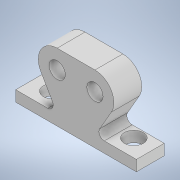
# Autodesk Inventor part: montaz_wachlarzy_2
Saved by Autodesk Inventor 2022 (Build 260153000, 153)
## iProperties
Created: 2022-12-26
Part Number: montaz_wachlarzy_2
Material: Generic
Document SubType Name: Modeling
Designer: Kamil
Density: 1 g/cm^3
Appearance: Default
Author: Kamil
Autodesk Inventor part; units mm, degrees
ref_plane "YZ Plane" through (0, 0, 0) normal (1, 0, 0) x (0, 1, 0)
ref_plane "XZ Plane" through (0, 0, 0) normal (0, 1, 0) x (-1, 0, 0)
ref_plane "XY Plane" through (0, 0, 0) normal (0, 0, 1) x (1, 0, 0)
sketch "Sketch1" plane through (0, 0, 0) normal (0, 0, 1) x (1, 0, 0)
  line L0 (28.1525, 7.6) -> (28.1525, 11.1) projected
  line L1 (-46.8475, 11.1) -> (28.1525, 11.1) projected
  line L2 (-46.8475, 11.1) -> (-46.8475, 7.6) projected
  line L3 (-46.8475, 7.6) -> (-22.3475, 7.6) projected
  line L4 (-22.3475, 0) -> (-22.3475, 7.6) projected
  line L5 (-22.3475, 0) -> (-18.695, 0) projected
  line L6 (-18.695, 0) -> (-18.695, 2.6) projected
  line L7 (-15, 2.6) -> (-18.695, 2.6) projected
  line L8 (-15, 0) -> (-15, 2.6) projected
  line L9 (-15, 0) -> (-3.695, 0) projected
  line L10 (-3.695, 0) -> (-3.695, 2.6) projected
  line L11 (0, 2.6) -> (-3.695, 2.6) projected
  line L12 (0, 0) -> (0, 2.6) projected
  line L13 (0, 0) -> (3.6525, 0) projected
  line L14 (3.6525, 0) -> (3.6525, 7.6) projected
  line L15 (3.6525, 7.6) -> (28.1525, 7.6) projected
  line L16 (-24.3475, 7.6) -> (-24.3475, 11.1) projected
  line L17 (5.6525, 7.6) -> (5.6525, 11.1) projected
  line L18 (-3.5975, 2.6) -> (-3.5975, 11.1)
  line L19 (-0.0975, 2.6) -> (-0.0975, 11.1)
  line L20 (-15.0975, 2.6) -> (-15.0975, 11.1)
  line L21 (-18.5975, 2.6) -> (-18.5975, 11.1)
  line L22 (-59.3475, 18.1) -> (-59.3475, 7.1) projected
  line L23 (-59.3475, 7.1) -> (-53.3475, 7.1) projected
  line L24 (-53.3475, 7.1) -> (-53.3475, 8.1) projected
  line L25 (-53.3475, 8.1) -> (-53.3475, 11.1) projected
  line L26 (-53.3475, 11.1) -> (-53.3475, 18.1) projected
  line L27 (-53.3475, 18.1) -> (-59.3475, 18.1) projected
  line L28 (-18.5975, 11.1) -> (-0.0975, 11.1)
  line L29 (-0.0975, 11.1) -> (-0.0975, 18.1)
  line L30 (-0.0975, 18.1) -> (-18.5975, 18.1)
  line L31 (-18.5975, 18.1) -> (-18.5975, 11.1)
  line L32 (-53.3475, 18.1) -> (10.0147, 18.1)
  circle A0 centre (-9.3475, 18.1) radius 3.5
  circle A1 centre (-9.3475, 18.1) radius 1.75
  line L33 (1.8262, 11.1) -> (-20.5213, 11.1)
  line L34 (-20.5213, 11.1) -> (-20.5213, 13.1)
  line L35 (-20.5213, 13.1) -> (-14.8475, 13.1)
  line L36 (1.8262, 13.1) -> (1.8262, 11.1)
  line L37 (-12.8475, 18.1) -> (-12.8475, 15.1)
  line L38 (-5.8475, 18.1) -> (-5.8475, 15.1)
  arc A2 (-14.8475, 13.1) -> (-12.8475, 15.1) centre (-14.8475, 15.1) ccw
  line L39 (-3.8475, 13.1) -> (1.8262, 13.1)
  arc A3 (-5.8475, 15.1) -> (-3.8475, 13.1) centre (-3.8475, 15.1) ccw
  point P0 (-5.8475, 13.1)
  dimension "d0" = 7
  dimension "d1" = 3.5
  dimension "d2" = 2
  dimension "d3" = 2
  dimension "d4" = 2
  constraints: 32 end point, 6 point on circle, 6 point on line, 6 tangent, 5 parallel, 4 centre point, 4 perpendicular, 4 vertical, 3 horizontal, 1 coincident, 10 other
  measures "d0" diameter of A0
  measures "d1" diameter of A1
  measures "d2" distance of L33.end L34.end
  measures "d3" radius of A2
  measures "d4" radius of A3
ref_plane "Work Plane1" through (-24.3475, 0, -5.16) normal (0, 0, -1) x (0, 1, 0)
extrude "Extrusion1" add sketch "Sketch1" against normal up to surface (5.16 mm away) contours L1 L29 L39 L36 | L1 L31 L35 A2 L37 A0 L38 A3 L39 L29 | L1 L34 L35 L31 | A0 L30 A1 | L30 A1 A0
sketch "Sketch2" plane through (-20.5213, 11.1, 0) normal (0, -1, 0) x (1, 0, 0)
  circle A0 centre (18.6738, -3.2) radius 1.75 projected
  circle A1 centre (3.6738, -3.2) radius 1.75 projected
  line L0 (-3.8262, -10.16) -> (-1.3262, -10.16) projected
  arc A2 (-1.3262, -10.16) -> (-1.3262, -5.16) centre (-1.3262, -7.66) ccw projected
  line L1 (-1.3262, -5.16) -> (-3.8262, -5.16) projected
  line L2 (-3.8262, -5.16) -> (-3.8262, -10.16) projected
  line L3 (23.6738, -10.16) -> (26.1738, -10.16) projected
  line L4 (26.1738, -10.16) -> (26.1738, -5.16) projected
  line L5 (26.1738, -5.16) -> (23.6738, -5.16) projected
  arc A3 (23.6738, -5.16) -> (23.6738, -10.16) centre (23.6738, -7.66) ccw projected
  line L6 (48.6738, 0) -> (48.6738, -46.6121) projected
  line L7 (48.6738, -46.6121) -> (26.0339, -46.6121) projected
  line L8 (26.0339, -46.6121) -> (26.0339, -30.5552) projected
  line L9 (26.0339, -30.5552) -> (14.0514, -9.5814) projected
  line L10 (14.0514, -9.5814) -> (8.2961, -9.5814) projected
  line L11 (8.2961, -9.5814) -> (-3.8262, -30.8) projected
  line L12 (-3.8262, -30.8) -> (-3.8262, -46.6121) projected
  line L13 (-3.8262, -46.6121) -> (-26.3262, -46.6121) projected
  line L14 (-26.3262, -46.6121) -> (-26.3262, 0) projected
  line L15 (-26.3262, 0) -> (48.6738, 0) projected
  line L16 (22.3475, -5.16) -> (16.6738, -5.16) projected
  line L17 (16.6738, 0) -> (16.6738, -5.16) projected
  line L18 (22.3475, 0) -> (16.6738, 0) projected
  line L19 (22.3475, 0) -> (22.3475, -5.16) projected
  circle A4 centre (3.6738, -3.2) radius 1.75 projected
  line L20 (5.6738, -5.16) -> (0, -5.16) projected
  line L21 (0, 0) -> (0, -5.16) projected
  line L22 (5.6738, 0) -> (0, 0) projected
  line L23 (5.6738, 0) -> (5.6738, -5.16) projected
  circle A5 centre (18.6738, -3.2) radius 1.75 projected
  circle A6 centre (3.6738, -3.2) radius 1.75 projected
  line L24 (14.0514, -9.5814) -> (22.3475, -5.16)
  line L25 (0, 0) -> (0, -5.16) projected
  line L26 (0, -5.16) -> (8.2961, -9.5814)
  point P0 (20.5213, 0)
  constraints: 4 end point
extrude "Extrusion2" add sketch "Sketch2" against normal up to surface (2 mm away) contours L17 L16 L24 L10 L26 L20 L23 L15
sketch "Sketch3" plane through (-20.5213, 11.1, 0) normal (0, -1, 0) x (1, 0, 0)
  circle A0 centre (3.6738, -3.2) radius 1.75 projected
  circle A1 centre (18.6738, -3.2) radius 1.75 projected
  point P0 (20.5213, 0)
extrude "Extrusion3" cut sketch "Sketch3" against normal blind 10
fillet "Fillet1" radius 2 1 edges at (-9.3475, 13.1, -5.16)
sketch "Sketch4" plane through (-3.8475, 13.1, 0) normal (0, 1, 0) x (1, 0, 0)
  line L0 (-11, 0) -> (-11, 7.16) projected
  line L1 (0, 7.16) -> (-11, 7.16) projected
  line L2 (0, 0) -> (0, 7.16) projected
  line L3 (5.6738, 0) -> (0, 0) projected
  line L4 (5.6738, 0) -> (5.6738, 5.16) projected
  line L5 (-2.6223, 9.5814) -> (5.6738, 5.16) projected
  line L6 (-8.3777, 9.5814) -> (-2.6223, 9.5814) projected
  line L7 (-16.6738, 5.16) -> (-8.3777, 9.5814) projected
  line L8 (-16.6738, 0) -> (-16.6738, 5.16) projected
  line L9 (-11, 0) -> (-16.6738, 0) projected
  circle A0 centre (-13, 3.2) radius 1.75 projected
  circle A1 centre (2, 3.2) radius 1.75 projected
  line L10 (2, 3.2) -> (5.2, 3.2)
  line L11 (-8.3777, 9.5814) -> (-2.6223, 9.5814) projected
  line L12 (-5.5, 9.5814) -> (-5.5, 7.6751)
  line L13 (5.2, 1.3525) -> (2, -0.495)
  line L14 (2, -0.495) -> (-1.2, 1.3525)
  line L15 (-1.2, 1.3525) -> (-1.2, 5.0475)
  line L16 (-1.2, 5.0475) -> (2, 6.895)
  line L17 (2, 6.895) -> (5.2, 5.0475)
  line L18 (5.2, 5.0475) -> (5.2, 1.3525)
  line L19 (-13, 3.2) -> (-16.2, 3.2)
  line L20 (-16.2, 5.0475) -> (-13, 6.895)
  line L21 (-13, 6.895) -> (-9.8, 5.0475)
  line L22 (-9.8, 5.0475) -> (-9.8, 1.3525)
  line L23 (-9.8, 1.3525) -> (-13, -0.495)
  line L24 (-13, -0.495) -> (-16.2, 1.3525)
  line L25 (-16.2, 1.3525) -> (-16.2, 5.0475)
  line L26 (-9, 0) -> (-9, 5.16) projected
  line L27 (-2, 0) -> (-2, 5.16) projected
  line L28 (0, 0) -> (0, 7.16) projected
  line L29 (-2.174, 0.4287) -> (0, 0.4287)
  line L30 (0, 0.4287) -> (0, 7.16)
  line L31 (0, 7.16) -> (-2.174, 7.16)
  line L32 (-2.174, 7.16) -> (-2.174, 0.4287)
  line L33 (0, 7.16) -> (-11, 7.16) projected
  line L34 (-11, 0) -> (-9, 0)
  line L35 (-9, 0) -> (-9, 7.16)
  line L36 (-9, 7.16) -> (-11, 7.16)
  line L37 (-11, 7.16) -> (-11, 0)
  line L38 (-2, 0) -> (-2, 5.16) projected
  line L39 (0, 0) -> (-2, 0) projected
  line L40 (0, 0) -> (0, 7.16) projected
  line L41 (-2, 5.16) -> (0, 7.16) projected
  line L42 (-11, 0) -> (-11, 7.16) projected
  line L43 (-9, 0) -> (-11, 0) projected
  line L44 (-9, 0) -> (-9, 5.16) projected
  line L45 (-11, 7.16) -> (-9, 5.16) projected
  point P0 (3.8475, 0)
  point P1 (-2, 0)
  point P2 (-2.174, 7.16)
  point P3 (-2, 0.4287)
  dimension "d12" = 3.2
  constraints: 46 end point, 4 parallel, 3 horizontal, 3 midpoint, 2 coincident, 2 perpendicular, 2 symmetric about line, 1 point on line, 1 vertical, 26 other
  measures "d12" distance of L10.start L10.end
extrude "Extrusion4" cut sketch "Sketch4" along normal blind 10 contours L0 L23 L22 L21 L45 L26 L34 | L0 L21 L22 L23 | L45 L1 L35 | L1 L41 L27 L29 L32 | L2 L16 L15 L14 L29 L27 L41 | L2 L14 L15 L16 | L29 L2 L39 L27
sketch "Sketch5" plane through (-5.8475, 13.1, 0) normal (0, 1, 0) x (1, 0, 0)
  line L0 (-0.174, 7.16) -> (-7, 7.16) projected
  line L1 (-0.174, 7.16) -> (-0.174, 0.4287) projected
  line L2 (-0.174, 0.4287) -> (0, 0.4287) projected
  line L3 (0, 0.4287) -> (0, 0) projected
  line L4 (7.6738, 0) -> (0, 0) projected
  line L5 (7.6738, 0) -> (7.6738, 5.16) projected
  line L6 (-0.6223, 9.5814) -> (7.6738, 5.16) projected
  line L7 (-6.3777, 9.5814) -> (-0.6223, 9.5814) projected
  line L8 (-14.6738, 5.16) -> (-6.3777, 9.5814) projected
  line L9 (-14.6738, 0) -> (-14.6738, 5.16) projected
  line L10 (-7, 0) -> (-14.6738, 0) projected
  line L11 (-7, 0) -> (-7, 7.16) projected
  circle A0 centre (-11, 3.2) radius 1.75 projected
  circle A1 centre (4, 3.2) radius 1.75 projected
  line L12 (0, 0) -> (0, 0.4287) projected
  line L13 (-14.6738, 0) -> (7.6738, 0) projected
  line L14 (0, 0.4287) -> (-0.174, 0.4287)
  line L15 (-0.174, 0.4287) -> (-0.174, 0)
  line L16 (-0.174, 0) -> (0, 0)
  line L17 (0, 0) -> (0, 0.4287)
  point P0 (5.8475, 0)
  constraints: 8 end point, 2 parallel, 1 horizontal, 1 perpendicular, 1 point on line
extrude "Extrusion5" cut sketch "Sketch5" along normal blind 10 contours L2 L3 L13 L15
sketch "Sketch6" plane through (0, 0, 0) normal (0, 0, 1) x (1, 0, 0)
  line L0 (-6.0216, 13.1) -> (-6.0216, 19.1899) projected
  arc A0 (-6.0216, 19.1899) -> (-12.8475, 18.1) centre (-9.3475, 18.1) ccw projected
  line L1 (-12.8475, 18.1) -> (-12.8475, 13.1) projected
  line L2 (-12.8475, 13.1) -> (-20.5213, 13.1) projected
  line L3 (-20.5213, 13.1) -> (-20.5213, 11.1) projected
  line L4 (-20.5213, 11.1) -> (1.8262, 11.1) projected
  line L5 (1.8262, 11.1) -> (1.8262, 13.1) projected
  line L6 (1.8262, 13.1) -> (-6.0216, 13.1) projected
  circle A1 centre (-9.3475, 18.1) radius 1.75 projected
  line L7 (-59.3475, 18.1) -> (-59.3475, 7.1) projected
  line L8 (-59.3475, 7.1) -> (-53.3475, 7.1) projected
  line L9 (-53.3475, 7.1) -> (-53.3475, 8.1) projected
  line L10 (-53.3475, 8.1) -> (-53.3475, 11.1) projected
  line L11 (-53.3475, 11.1) -> (-53.3475, 18.1) projected
  line L12 (-53.3475, 18.1) -> (-59.3475, 18.1) projected
  line L13 (-9.3475, 18.1) -> (-9.3475, 20.1)
  circle A2 centre (-9.3475, 20.1) radius 1.75
  circle A3 centre (-9.3475, 20.1) radius 3.5
  line L14 (-6.4698, 13.1) -> (1.8262, 13.1) projected
  line L15 (-12.8475, 20.1) -> (-5.8475, 20.1)
  line L16 (-5.8475, 20.1) -> (-5.8475, 13.1)
  line L17 (-5.8475, 13.1) -> (-12.8475, 13.1)
  line L18 (-12.8475, 13.1) -> (-12.8475, 20.1)
  point P0 (0, 0)
  point P1 (-12.8475, 18.1)
  dimension "d17" = 2
  constraints: 10 end point, 2 coincident, 2 parallel, 1 centre point, 1 horizontal, 1 perpendicular, 1 point on line, 1 vertical, 3 other
  measures "d17" distance of L13.start L13.end
extrude "Extrusion6" add sketch "Sketch6" against normal up to surface (5.16 mm away) contours L14 L17 L1 A0 A3 A1 L0 | L0 A3 L16 L6 | A3 A1 A2 L15 A0 L0 | L0 A0 L15 A3 | A3 A1 A2 | A1 A3 | L15 A0 A2 A3 | L15 A2 A0 | A3 A0 L15 A2 A1 | L15 A0 A3 | A3 A0 L18 | A2 L15 A0 | A0 A2 | A2 A1 L13 L15 | A2 L15 L13 A1 | A1 L13 A2 | A2 L13 A1 | A0 A2 L15
sketch "Sketch7" plane through (0, 0, 0) normal (0, 0, 1) x (1, 0, 0)
  line L0 (-12.8475, 13.1) -> (-20.5213, 13.1) projected
  line L1 (-20.5213, 13.1) -> (-20.5213, 11.1) projected
  line L2 (-20.5213, 11.1) -> (1.8262, 11.1) projected
  line L3 (1.8262, 11.1) -> (1.8262, 13.1) projected
  line L4 (1.8262, 13.1) -> (-5.8475, 13.1) projected
  line L5 (-5.8475, 13.1) -> (-5.8475, 20.1) projected
  arc A0 (-5.8475, 20.1) -> (-12.8475, 20.1) centre (-9.3475, 20.1) ccw projected
  line L6 (-12.8475, 20.1) -> (-12.8475, 13.1) projected
  circle A1 centre (-9.3475, 20.1) radius 1.75
  point P0 (0, 0)
  dimension "d20" = 3.5
  constraints: 1 centre point, 1 coincident
  measures "d20" diameter of A1
extrude "Extrusion7" cut sketch "Sketch7" against normal blind 10 contours A1
sketch "Sketch8" plane through (0, 0, 0) normal (0, 0, 1) x (1, 0, 0)
  circle A0 centre (-9.3475, 20.1) radius 1.75 projected
  line L0 (-12.8475, 13.1) -> (-20.5213, 13.1) projected
  line L1 (-20.5213, 13.1) -> (-20.5213, 11.1) projected
  line L2 (-20.5213, 11.1) -> (1.8262, 11.1) projected
  line L3 (1.8262, 11.1) -> (1.8262, 13.1) projected
  line L4 (1.8262, 13.1) -> (-5.8475, 13.1) projected
  line L5 (-5.8475, 13.1) -> (-5.8475, 20.1) projected
  arc A1 (-5.8475, 20.1) -> (-12.8475, 20.1) centre (-9.3475, 20.1) ccw projected
  line L6 (-12.8475, 20.1) -> (-12.8475, 13.1) projected
  circle A2 centre (-9.3475, 20.1) radius 3.5
  arc A3 (-5.8475, 20.1) -> (-12.8475, 20.1) centre (-9.3475, 20.1) ccw projected
  circle A4 centre (-5.8475, 20.1) radius 1.5
  line L7 (-12.8475, 20.1) -> (-12.8475, 15.1) projected
  circle A5 centre (-12.8475, 20.1) radius 1.5
  line L8 (-5.8475, 13.1) -> (-5.8475, 20.1) projected
  circle A6 centre (-5.8475, 20.1) radius 3.5
  circle A7 centre (-12.8475, 20.1) radius 3.5
  line L9 (-12.8475, 13.1) -> (-15.8786, 18.35)
  line L10 (-5.8475, 13.1) -> (-2.8164, 18.35)
  line L11 (-12.8475, 23.6) -> (-5.8475, 23.6)
  line L12 (-12.2252, 13.1) -> (-6.4698, 13.1) projected
  point P0 (0, 0)
  point P1 (-9.3475, 23.6)
  point P2 (-12.8475, 18.6)
  point P3 (-12.5261, 21.5652)
  point P4 (-6.1689, 21.5652)
  point P5 (-5.8475, 18.6)
  dimension "d23" = 3
  dimension "d24" = 3
  constraints: 7 point on circle, 6 end point, 4 centre point, 4 coincident, 3 tangent, 1 horizontal alignment, 1 parallel, 2 other
  measures "d23" diameter of A4
  measures "d24" diameter of A5
extrude "Extrusion8" add sketch "Sketch8" against normal up to surface (5.16 mm away) contours A0 A6 | A6 A7 A0 | A0 A7 A6 | A7 A0 | A6 L5 A4 A1 | A1 L11 A6 | A7 L11 A1 | A1 A5 L6 A7 | A6 L10 L5 | L6 L9 A7
extrude "Extrusion9" cut sketch "Sketch8" against normal through all contours A1 A2 A4 | A2 L5 A4 | A5 A2 A1 | A1 L6 A5 | A5 L6 A2
fillet "Fillet2" radius 1 2 edges at (-5.8475, 13.1, -2.58) (-12.8475, 13.1, -2.58)
sketch "Sketch9" plane through (-6.0216, 13.1, -5.16) normal (1, 0, 0) x (0, 0, -1)
  line L0 (0, 2) -> (0, 0) projected
  line L1 (2, 0) -> (0, 0) projected
  arc A0 (0, 2) -> (2, 0) centre (2, 2) ccw projected
  point P0 (-5.16, -13.1)
extrude "Extrusion10" cut sketch "Sketch9" against normal blind 10
sketch "Sketch10" plane through (-12.2252, 13.1, -9.5814) normal (0, 1, 0) x (1, 0, 0)
  line L0 (-2.3544, -4.4214) -> (8.1097, -4.4214) projected
  line L1 (8.1097, -9.5814) -> (8.1097, -4.4214) projected
  line L2 (14.0514, -9.5814) -> (8.1097, -9.5814) projected
  line L3 (14.0514, -9.5814) -> (14.0514, -4.4214) projected
  line L4 (5.7554, 0) -> (14.0514, -4.4214) projected
  line L5 (0, 0) -> (5.7554, 0) projected
  line L6 (-8.2961, -4.4214) -> (0, 0) projected
  line L7 (-8.2961, -9.5814) -> (-8.2961, -4.4214) projected
  line L8 (-2.3544, -9.5814) -> (-8.2961, -9.5814) projected
  line L9 (-2.3544, -4.4214) -> (-2.3544, -9.5814) projected
  circle A0 centre (-4.6223, -6.3814) radius 1.75 projected
  circle A1 centre (10.3777, -6.3814) radius 1.75 projected
  line L10 (-8.2961, -9.5814) -> (14.0514, -9.5814) projected
  line L11 (-8.2961, -4.4214) -> (0, 0) projected
  line L12 (14.0514, -9.5814) -> (-8.2961, -9.5814)
  line L13 (-8.2961, -9.5814) -> (-8.2961, -4.4214)
  line L14 (-8.2961, -4.4214) -> (14.0514, -4.4214)
  line L15 (14.0514, -4.4214) -> (14.0514, -9.5814)
  point P0 (12.2252, -9.5814)
  point P1 (-2.3544, -4.4214)
  constraints: 8 end point, 2 parallel, 1 horizontal, 1 perpendicular
extrude "Extrusion11" cut sketch "Sketch10" against normal blind 10 contours L14 L6 L5 L4 L0
body "Solid1"
